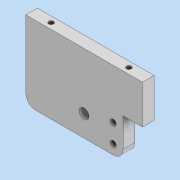
# Autodesk Inventor part: X-Axis_beltplates
Saved by Autodesk Inventor 2022 (Build 260153000, 153)
## iProperties
Created: 2021-04-15
Part Number: X-Axis_beltplates
Material: Generic
Document SubType Name: Modeling
Designer: Fabijan_Sven
Density: 1 g/cm^3
Appearance: Default
Author: Fabijan_Sven
Autodesk Inventor part; units mm, degrees
ref_plane "YZ Plane" through (0, 0, 0) normal (1, 0, 0) x (0, 1, 0)
ref_plane "XZ Plane" through (0, 0, 0) normal (0, 1, 0) x (-1, 0, 0)
ref_plane "XY Plane" through (0, 0, 0) normal (0, 0, 1) x (1, 0, 0)
sketch "Sketch1" plane through (0, 0, 0) normal (0, 1, 0) x (-1, 0, 0)
  line L0 (0, 0) -> (60, 0)
  line L1 (60, 0) -> (60, -6)
  line L2 (60, -6) -> (0, -6)
  line L3 (0, -6) -> (0, 0)
  dimension "d7" = 60
  dimension "d8" = 6
  constraints: 8 end point, 2 parallel, 1 horizontal, 1 perpendicular
  measures "d7" distance of L1.end L2.end
  measures "d8" distance of L0.end L1.end
extrude "Extrusion1" add sketch "Sketch1" along normal blind 40
sketch "Sketch2" plane through (0, 0, -6) normal (0, 0, -1) x (-1, 0, 0)
  circle A0 centre (30, 11) radius 2.5
  line L0 (0, 40) -> (60, 40) projected
  line L1 (0, 0) -> (0, 40) projected
  line L2 (0, 0) -> (60, 0) projected
  dimension "d2" = 5
  dimension "d3" = 29
  dimension "d4" = 30
  constraints: 1 centre point
  measures "d2" diameter of A0
  measures "d3" distance from line of L0 A0.centre
  measures "d4" distance from line of L1 A0.centre
extrude "Extrusion2" cut sketch "Sketch2" against normal blind 10
fillet "Fillet1" radius 5 2 edges at (-60, 0, -3) (0, 0, -3)
sketch "Sketch3" plane through (-60, 40, 0) normal (0, 0, 1) x (1, 0, 0)
  circle A0 centre (45, -35) radius 1.5
  circle A1 centre (45, -25.5) radius 1.5
  line L0 (5, -40) -> (55, -40) projected
  line L1 (60, -35) -> (60, 0) projected
  point P0 (60, -40)
  dimension "d16" = 5
  dimension "d17" = 9.5
  dimension "d18" = 15
  dimension "d20" = 3
  dimension "d21" = 3
  dimension "d42" = 15
  constraints: 2 centre point
  measures "d16" distance from line of L0 A0.centre
  measures "d17" distance of A1.centre A0.centre
  measures "d18" distance from line of L1 A1.centre
  measures "d20" diameter of A0
  measures "d21" diameter of A1
  measures "d42" distance from line of L1 A0.centre
hole "Hole1" at (-15, 5, 0) at (-15, 14.5, 0) direction (0, 0, -1) diameter 3 end through all
sketch "Sketch4" plane through (0, 40, 0) normal (0, 1, 0) x (1, 0, 0)
  circle A0 centre (-10, 2.5) radius 1.5 projected
  circle A1 centre (-50, 2.5) radius 1.5 projected
  circle A2 centre (-50, 3) radius 1.5
  circle A3 centre (-10, 3) radius 1.5
  line L0 (-60, 0) -> (0, 0) projected
  line L1 (-60, 6) -> (-60, 0) projected
  line L2 (0, 0) -> (0, 6) projected
  dimension "d36" = 3
  dimension "d37" = 3
  dimension "d38" = 10
  dimension "d39" = 10
  dimension "d40" = 3
  dimension "d41" = 3
  constraints: 2 centre point
  measures "d36" distance from line of L0 A2.centre
  measures "d37" distance from line of L0 A3.centre
  measures "d38" distance from line of L1 A2.centre
  measures "d39" distance from line of A3.centre L2
  measures "d40" diameter of A3
  measures "d41" diameter of A2
hole "Hole2" at (-50, 40, -3) at (-10, 40, -3) direction (0, -1, 0) diameter 2.459 depth 8.8 tip angle 118 thread size "M3x0.5" class "6H" standard "ISO Metric profile"
sketch "Sketch5" plane through (-60, 40, 0) normal (0, 0, 1) x (1, 0, 0)
  line L0 (70, -50) -> (50, -50)
  line L1 (50, -50) -> (50, -20)
  line L2 (50, -20) -> (70, -20)
  line L3 (70, -20) -> (70, -50)
  line L4 (5, -40) -> (55, -40) projected
  line L5 (60, -35) -> (60, 0) projected
  point P0 (60, -40)
  dimension "d43" = 10
  dimension "d44" = 10
  dimension "d45" = 20
  dimension "d46" = 10
  constraints: 8 end point, 2 parallel, 1 horizontal, 1 perpendicular
  measures "d43" distance between parallel lines of L4 L0
  measures "d44" distance between parallel lines of L5 L1
  measures "d45" distance between parallel lines of L4 L2
  measures "d46" distance between parallel lines of L5 L3
extrude "Extrusion3" cut sketch "Sketch5" against normal blind 10
fillet "Fillet2" radius 5 1 edges at (-10, 0, -3)
equation "\"d22\" = d20"
body "Solid1"
